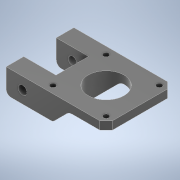
# Autodesk Inventor part: Zmotorsupport
Saved by Autodesk Inventor 2022 (Build 260153000, 153)
## iProperties
Created: 2022-02-20
Part Number: Zmotorsupport
Material: Genérico
Document SubType Name: Modeling
Designer: JK
Density: 1 g/cm^3
Appearance: Suave - Negro
Author: JK
Autodesk Inventor part; units mm, degrees
ref_plane "YZ Plane" through (0, 0, 0) normal (1, 0, 0) x (0, 1, 0)
ref_plane "XZ Plane" through (0, 0, 0) normal (0, 1, 0) x (-1, 0, 0)
ref_plane "XY Plane" through (0, 0, 0) normal (0, 0, 1) x (1, 0, 0)
sketch "Boceto1" plane through (0, 0, 0) normal (0, 1, 0) x (-1, 0, 0)
  line L0 (-21, 21) -> (21, 21)
  line L1 (21, 21) -> (21, -21)
  line L2 (21, -21) -> (-21, -21)
  line L3 (-21, -21) -> (-21, 21)
  line L4 (-21, 21) -> (21, -21) construction
  line L5 (21, 21) -> (-21, -21) construction
  circle A0 centre (0, 0) radius 11.1
  dimension "d0" = 42
  dimension "d1" = 42
  dimension "d2" = 22.2
  constraints: 12 end point, 2 midpoint, 2 parallel, 1 centre point, 1 coincident, 1 horizontal, 1 perpendicular
  measures "d0" distance of L0.end L1.end
  measures "d1" distance of L1.end L2.end
  measures "d2" diameter of A0
extrude "Extrusión1" add sketch "Boceto1" along normal blind 5
sketch "Boceto3" plane through (0, 0, 0) normal (0, -1, 0) x (1, 0, 0)
  circle A0 centre (16.5, 16.5) radius 1.65
  point P0 (0, 0)
  dimension "d9" = 3.3
  dimension "d10" = 16.5
  dimension "d11" = 16.5
  constraints: 1 centre point
  measures "d9" diameter of A0
  measures "d10" horizontal distance of point (0, 0) A0.centre
  measures "d11" horizontal distance of A0.centre point (0, 0)
extrude "Extrusión3" cut sketch "Boceto3" against normal through all
chamfer "Chaflán1" distance 1.5 angle 45 1 edges at (14.85, 0, 16.5)
pattern_circular "Patrón circular1" count 4 over 360 about axis through (0, 0, 0) along (0, 1, 0) of "Extrusión3", "Chaflán1"
chamfer "Chaflán3" distance 4 angle 45 2 edges at (21, 2.5, -21) (21, 2.5, 21)
sketch "Boceto4" plane through (0, 0, 0) normal (0, -1, 0) x (1, 0, 0)
  circle A0 centre (-16.5, 16.5) radius 3.15 projected
  circle A1 centre (-16.5, 16.5) radius 1.65 projected
  circle A2 centre (-16.5, -16.5) radius 1.65 projected
  circle A3 centre (-16.5, -16.5) radius 3.15 projected
  line L0 (-21, -21) -> (-21, 21) projected
  line L1 (17, -21) -> (-21, -21) projected
  line L2 (-21, 21) -> (-12, 21)
  line L3 (-12, 21) -> (-12, -21)
  line L4 (-12, -21) -> (-21, -21)
  line L5 (-21, -21) -> (-21, 21)
  point P0 (0, 0)
  dimension "d27" = 9
  constraints: 8 end point, 2 parallel, 1 horizontal, 1 perpendicular, 1 point on line
  measures "d27" distance between parallel lines of L3 L0
extrude "Extrusión4" add sketch "Boceto4" along normal blind 10 contours L0 L2 L3 L1
sketch "Boceto5" plane through (0, -10, 0) normal (0, -1, 0) x (1, 0, 0)
  line L0 (-21, -21) -> (-21, 21) projected
  line L1 (-21, 21) -> (-41, 21)
  line L2 (-41, 21) -> (-41, -21)
  line L3 (-41, -21) -> (-21, -21)
  line L4 (-21, -21) -> (-21, 21)
  line L5 (-21, 10.1) -> (-41, 10.1)
  line L6 (-41, 10.1) -> (-41, -10.1)
  line L7 (-41, -10.1) -> (-21, -10.1)
  line L8 (-21, -10.1) -> (-21, 10.1)
  line L9 (-31, 10.1) -> (-31, 21)
  line L10 (-31, -10.1) -> (-31, -21)
  line L11 (-21, -21) -> (-12, -21) projected
  point P0 (0, 0)
  dimension "d30" = 20.2
  dimension "d31" = 20
  constraints: 20 end point, 4 midpoint, 4 parallel, 2 collinear, 2 horizontal, 2 perpendicular, 2 point on line
  measures "d30" distance between parallel lines of L7 L5
  measures "d31" distance between parallel lines of L2 L0
extrude "Extrusión5" add sketch "Boceto5" against normal up to surface (15 mm away) contours L3 L10 L7 L0 | L3 L2 L7 L10 | L5 L9 L1 L0 | L5 L2 L1 L9
chamfer "Chaflán4" distance 10 angle 45 1 edges at (-12, 0, 0)
fillet "Empalme2" radius 5 2 edges at (-2, 0, -15.9592) (-2, 0, 15.9592)
fillet "Empalme3" radius 3 1 edges at (-12, -10, 0)
fillet "Empalme4" radius 3 2 edges at (-41, -10, 15.55) (-41, -10, -15.55)
sketch "Boceto6" plane through (17, 0, -21) normal (0, 0, -1) x (-1, 0, 0)
  circle A0 centre (47.9, -2.5) radius 2.65
  line L0 (0, 5) -> (58, 5) projected
  line L1 (58, -7) -> (58, 5) projected
  point P0 (17, 0)
  dimension "d40" = 7.5
  dimension "d41" = 10.1
  dimension "d42" = 5.3
  constraints: 1 centre point
  measures "d40" distance from line of L0 A0.centre
  measures "d41" distance from line of L1 A0.centre
  measures "d42" diameter of A0
extrude "Extrusión6" cut sketch "Boceto6" against normal through all
